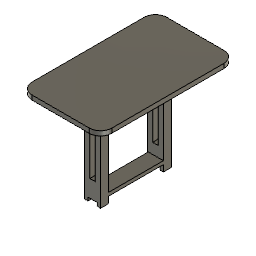
blimp-gondola-mount (Autodesk Fusion 360 design; units mm, degrees)
Autodesk Fusion 360 part; units mm, degrees
sketch "Sketch1" plane through (0, 0, 0) normal (0, 0, 1) x (1, 0, 0)
  line L0 (-3.5, -2.6546) -> (3.5, -2.6546)
  line L1 (3.5, -2.6546) -> (3.5, 0.8454)
  line L2 (3.5, 0.8454) -> (-3.5, 0.8454)
  line L3 (-3.5, 0.8454) -> (-3.5, -2.6546)
  circle A0 centre (0, -0.9046) radius 1
  line L4 (-6.5474, 12.8454) -> (3.4526, 12.8454) construction
  line L5 (-3.5, 28.3454) -> (3.5, 28.3454)
  line L6 (-3.5, 24.8454) -> (-3.5, 28.3454)
  circle A1 centre (0, 26.5954) radius 1
  line L7 (3.5, 28.3454) -> (3.5, 24.8454)
  line L8 (3.5, 24.8454) -> (-3.5, 24.8454)
  line L9 (-2, 0.8454) -> (2, 0.8454)
  line L10 (2, 0.8454) -> (2, -2.6546)
  line L11 (2, -2.6546) -> (-2, -2.6546)
  line L12 (-2, -2.6546) -> (-2, 0.8454)
  line L13 (-2, 0.8454) -> (2, -2.6546) construction
  line L14 (2, 0.8454) -> (-2, -2.6546) construction
  line L15 (-2, 28.3454) -> (-2, 24.8454)
  line L16 (2, 24.8454) -> (2, 28.3454)
  line L17 (2, 28.3454) -> (-2, 28.3454)
  line L18 (-2, 24.8454) -> (2, 24.8454)
  point P0 (0, 0.8454)
  point P1 (3.5, -0.9046)
  point P2 (3.5, 26.5954)
  point P3 (0, 24.8454)
  point P4 (0, 25.6909)
  point P5 (0, -0.9046)
  dimension "d1" = 2
  dimension "d2" = 3.5
  dimension "d3" = 7
  dimension "d4" = 10
  dimension "d5" = 12
  dimension "d30" = 4
  constraint horizontal L0
  constraint vertical L1
  constraint horizontal L2
  constraint vertical L3
  constraint midpoint L2 P0
  constraint vertical origin P0
  constraint midpoint L1 P1
  constraint horizontal P5 P1
  constraint horizontal L4
  constraint symmetric origin L4 P4
  constraint symmetric L0.start L4 L5.start
  constraint symmetric L0.end L4 L5.end
  constraint symmetric L1.end L4 L7.end
  constraint symmetric L2.end L4 L6.start
  constraint symmetric P0 L4 P3
  constraint symmetric A0 L4 A1
  constraint symmetric P1 L4 P2
  constraint horizontal L9
  constraint perpendicular L9 L10
  constraint parallel L9 L11
  constraint parallel L10 L12
  constraint coincident L13 P5
  constraint coincident L14 P5
  constraint coincident L2 L9.start
  constraint coincident P5 A0.centre
  constraint symmetric L4 L9.start L15.end
  constraint symmetric L4 L9.end L16.start
  constraint symmetric L4 L10.end L16.end
  constraint symmetric L4 L11.end L15.start
  measures "d1" diameter of A0
  measures "d2" distance of L0.end L1.end
  measures "d3" distance of L1.end L2.end
  measures "d4" distance of L4.start L4.end
  measures "d5" distance of L2 L4
  measures "d30" distance of L10 L12
extrude "Extrude1" add sketch "Sketch1" along normal blind 40 contours L0 L2 L3 L12 | L0 L2 L9 L10 L11 L12 | L0 L1 L2 L10 | A0 | L5 L6 L8 L15 | L5 L8 L15 L16 L17 L18 | L5 L7 L8 L16 | A1 makes body 1 at (1.1667, 0.8454, 13.3333) makes body 2 at (-1.1667, 28.3454, 13.3333)
extrude "Extrude2" cut sketch "Sketch1" along normal blind 8 contours A0 | A1 bodies 1 2
sketch "Sketch2" plane through (0, 0.8454, 0) normal (0, 1, 0) x (-1, 0, 0)
  line L0 (-3.5, 0) -> (3.5, 0)
  line L1 (3.5, 0) -> (3.5, 40)
  line L2 (3.5, 40) -> (-3.5, 40)
  line L3 (-3.5, 40) -> (-3.5, 0)
  line L4 (-1.2, 37) -> (1.2, 37)
  line L5 (1.2, 37) -> (1.2, 9)
  line L6 (1.2, 9) -> (-1.2, 9)
  line L7 (-1.2, 9) -> (-1.2, 37)
  line L8 (3.5, 0) -> (-3.5, 0)
  dimension "d10" = 2.3
  dimension "d11" = 2.3
  dimension "d12" = 9
  dimension "d13" = 3
  constraint horizontal L4
  constraint vertical L5
  constraint horizontal L6
  constraint vertical L7
  measures "d10" distance of L1 L5
  measures "d11" distance of L3 L7
  measures "d12" distance of L6 L8
  measures "d13" distance of L2 L4
extrude "Extrude3" cut sketch "Sketch2" along normal through all and the other way through all contours L4 L5 L6 L7 bodies 2
sketch "Sketch3" plane through (0, 0, 0) normal (0, 0, 1) x (1, 0, 0)
  line L0 (17.5, -16.6546) -> (-17.5, -16.6546)
  line L1 (-17.5, -16.6546) -> (-17.5, 42.3454)
  line L2 (-17.5, 42.3454) -> (17.5, 42.3454)
  line L3 (17.5, 42.3454) -> (17.5, -16.6546)
  line L4 (-3.5, -2.6546) -> (3.5, -2.6546)
  line L5 (-3.5, 0.8454) -> (-3.5, -2.6546)
  line L6 (-3.5, 28.3454) -> (3.5, 28.3454)
  line L7 (-4, -16.6546) -> (4, -16.6546)
  line L8 (4, -16.6546) -> (4, -34.6546)
  line L9 (4, -34.6546) -> (-4, -34.6546)
  line L10 (-4, -34.6546) -> (-4, -16.6546)
  line L11 (-4, 42.3454) -> (4, 42.3454)
  line L12 (4, 42.3454) -> (4, 60.3454)
  line L13 (4, 60.3454) -> (-4, 60.3454)
  line L14 (-4, 60.3454) -> (-4, 42.3454)
  line L15 (17.5, 8.8454) -> (35.5, 8.8454)
  line L16 (35.5, 8.8454) -> (35.5, 16.8454)
  line L17 (35.5, 16.8454) -> (17.5, 16.8454)
  line L18 (17.5, 16.8454) -> (17.5, 8.8454)
  line L19 (-17.5, 8.8454) -> (-35.5, 8.8454)
  line L20 (-35.5, 8.8454) -> (-35.5, 16.8454)
  line L21 (-35.5, 16.8454) -> (-17.5, 16.8454)
  line L22 (-17.5, 16.8454) -> (-17.5, 8.8454)
  point P0 (3.5, -0.9046)
  point P1 (0, -34.6546)
  point P2 (-35.5, 12.8454)
  point P3 (35.5, 12.8454)
  point P4 (0, 60.3454)
  point P5 (-17.5, 12.8454)
  dimension "d15" = 14
  dimension "d16" = 14
  dimension "d17" = 14
  dimension "d18" = 14
  dimension "d43" = 8
  dimension "d44" = 18
  constraint horizontal L0
  constraint vertical L1
  constraint horizontal L2
  constraint vertical L3
  constraint horizontal L7
  constraint vertical L8
  constraint horizontal L9
  constraint vertical L10
  constraint coincident L0 L7.start
  constraint horizontal L11
  constraint vertical L12
  constraint horizontal L13
  constraint vertical L14
  constraint coincident L2 L11.start
  constraint horizontal L15
  constraint vertical L16
  constraint horizontal L17
  constraint vertical L18
  constraint coincident L3 L15.start
  constraint horizontal L19
  constraint vertical L20
  constraint horizontal L21
  constraint vertical L22
  constraint coincident L1 L19.start
  constraint equal L17 L19
  constraint equal L12 L17
  constraint equal L8 L17
  constraint equal L9 L20
  constraint equal L16 L20
  constraint equal L13 L16
  constraint midpoint L9 P1
  constraint midpoint L20 P2
  constraint midpoint L16 P3
  constraint midpoint L13 P4
  constraint vertical origin P4
  constraint vertical origin P1
  constraint midpoint L1 P5
  constraint horizontal P2 P5
  constraint horizontal P3 P5
  measures "d15" distance of L0 L4
  measures "d16" distance of L1 L5
  measures "d17" distance of L3 P0
  measures "d18" distance of L2 L6
  measures "d43" distance of L15.end L16.end
  measures "d44" distance of L7.end L8.end
extrude "Extrude4" add sketch "Sketch3" along normal blind 2 from surface at 40 contours L0 L1 L2 L3 L7 L11 L18 L22 bodies 1 2
fillet "Fillet1" radius 5 4 edges at (-17.5, -16.6546, 41) (-17.5, 42.3454, 41) (17.5, 42.3454, 41) (17.5, -16.6546, 41) on bodies 1
fillet "Fillet1" radius 2 8 edges at (0, 28.3454, 40) (-3.5, 26.5954, 40) (3.5, 26.5954, 40) (0, 24.8454, 40) (3.5, -0.9046, 40) (0, -2.6546, 40) (-3.5, -0.9046, 40) (0, 0.8454, 40) on bodies 1
extrude "Extrude5" cut sketch "Sketch2" against normal blind 8 contours L4 L5 L6 L7 bodies 1
extrude "Extrude6" cut sketch "Sketch1" along normal blind 1.5 contours L0 L2 L9 L10 L11 L12 | L5 L8 L15 L16 L17 L18 bodies 1
sketch "Sketch4" plane through (0, 24.8454, 0) normal (0, -1, 0) x (1, 0, 0)
  line L0 (-1.2, 9) -> (-1.2, 37)
  line L1 (-1.2, 37) -> (1.2, 37)
  line L2 (1.2, 37) -> (1.2, 9)
  line L3 (1.2, 9) -> (-1.2, 9)
  line L4 (-2, 0) -> (-2, 1.5)
  line L5 (-2, 1.5) -> (2, 1.5)
  line L6 (2, 1.5) -> (2, 0)
  line L7 (2, 0) -> (3.5, 0)
  line L8 (3.5, 0) -> (3.5, 38)
  line L9 (3.5, 38) -> (-3.5, 38)
  line L10 (-3.5, 38) -> (-3.5, 0)
  line L11 (-3.5, 0) -> (-2, 0)
  line L12 (3.5, 4.35) -> (-3.5, 4.35)
  line L13 (-3.5, 4.35) -> (-3.5, 2.85)
  line L14 (-3.5, 2.85) -> (3.5, 2.85)
  line L15 (3.5, 2.85) -> (3.5, 4.35)
  line L16 (-3.5, 2.85) -> (-3.1607, 2.85)
  line L17 (-3.1607, 2.85) -> (-3.1607, 4.35)
  line L18 (-3.1607, 4.35) -> (-3.5, 4.35)
  line L19 (-3.5, 4.35) -> (-3.5, 2.85)
  point P0 (3.5, 0)
  dimension "d40" = 1.5
  dimension "d42" = 2.85
  constraint horizontal L12
  constraint vertical L13
  constraint horizontal L14
  constraint vertical L15
  constraint coincident L10 L13.end
  constraint vertical P0 L14.end
  constraint horizontal L16
  constraint vertical L17
  constraint horizontal L18
  constraint vertical L19
  constraint coincident L12 L17.end
  measures "d40" distance of L12.start L14.end
  measures "d42" distance of L10.end L13.end
extrude "Extrude7" add sketch "Sketch4" along normal up to surface (24 mm away) contours L8 L12 L14 L15 L17 bodies 1
equation "d11 = d10"
equation "d16 = d15"
equation "d17 = d16"
equation "d18 = d15"
equation "d34 = 1.5 mm"
equation "d40 = d34"
